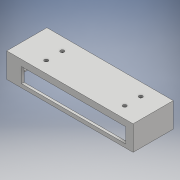
# Autodesk Inventor part: usbhub_holder_new
Saved by Autodesk Inventor 2018 (Build 220112000, 112)
## iProperties
Created: 2019-07-27
Part Number: usbhub_holder_new
Material: 一般
Document SubType Name: Modeling
Designer: guest1
Density: 1 g/cm^3
Appearance: 既定
Author: guest1
Autodesk Inventor part; units mm, degrees
ref_plane "YZ Plane" through (0, 0, 0) normal (1, 0, 0) x (0, 1, 0)
ref_plane "XZ Plane" through (0, 0, 0) normal (0, 1, 0) x (-1, 0, 0)
ref_plane "XY Plane" through (0, 0, 0) normal (0, 0, 1) x (1, 0, 0)
sketch "スケッチ1" plane through (0, 0, 0) normal (0, 0, 1) x (1, 0, 0)
  line L0 (52.125, -16.25) -> (-52.125, -16.25)
  line L1 (-52.125, -16.25) -> (-52.125, 16.25)
  line L2 (-52.125, 16.25) -> (52.125, 16.25)
  line L3 (52.125, 16.25) -> (52.125, -16.25)
  line L4 (52.125, -16.25) -> (-52.125, 16.25) construction
  line L5 (-52.125, -16.25) -> (52.125, 16.25) construction
  point P0 (0, 0)
  dimension "d0" = 104.25
  dimension "d1" = 32.5
  constraints: 12 end point, 2 midpoint, 2 parallel, 1 horizontal, 1 perpendicular
  measures "d0" distance of L1.end L2.end
  measures "d1" distance of L2.end L0.start
extrude "枠" add sketch "スケッチ1" along normal blind 19
sketch "スケッチ2" plane through (0, 0, 0) normal (0, 0, -1) x (-1, 0, 0)
  line L0 (50.125, -14.25) -> (-50.125, -14.25)
  line L1 (-50.125, -14.25) -> (-50.125, 14.25)
  line L2 (-50.125, 14.25) -> (50.125, 14.25)
  line L3 (50.125, 14.25) -> (50.125, -14.25)
  line L4 (50.125, -14.25) -> (-50.125, 14.25) construction
  line L5 (-50.125, -14.25) -> (50.125, 14.25) construction
  point P0 (0, 0)
  dimension "d4" = 100.25
  dimension "d5" = 28.5
  constraints: 12 end point, 2 midpoint, 2 parallel, 1 horizontal, 1 perpendicular
  measures "d4" distance of L1.end L2.end
  measures "d5" distance between parallel lines of L2 L0
extrude "本体" cut sketch "スケッチ2" against normal blind 12
sketch "スケッチ3" plane through (-52.125, -16.25, 0) normal (-1, 0, 0) x (0, 0, 1)
  line L0 (2, 2) -> (14, 2)
  line L1 (14, 2) -> (14, 30.5)
  line L2 (14, 30.5) -> (2, 30.5)
  line L3 (2, 30.5) -> (2, 2)
  line L4 (19, 32.5) -> (19, 0) projected
  line L5 (0, 0) -> (19, 0) projected
  line L6 (0, 0) -> (0, 32.5) projected
  line L7 (0, 32.5) -> (19, 32.5) projected
  point P0 (0, 16.25)
  dimension "d8" = 5
  dimension "d9" = 28.5
  dimension "d10" = 2
  dimension "d11" = 12
  dimension "d12" = 2
  dimension "d13" = 2
  constraints: 8 end point, 2 parallel, 1 horizontal, 1 perpendicular
  measures "d8" distance between parallel lines of L4 L1
  measures "d9" distance of L2.end L0.start
  measures "d10" distance between parallel lines of L5 L0
  measures "d11" distance of L1.end L2.end
  measures "d12" distance between parallel lines of L3 L6
  measures "d13" distance between parallel lines of L7 L2
extrude "入口" cut sketch "スケッチ3" against normal blind 102.25 contours L3 L2 L1 L0
sketch "スケッチ4" plane through (-52.125, -16.25, 0) normal (0, -1, 0) x (1, 0, 0)
  line L0 (98.25, 2) -> (14, 2)
  line L1 (14, 2) -> (14, 14)
  line L2 (14, 14) -> (98.25, 14)
  line L3 (98.25, 14) -> (98.25, 2)
  line L4 (104.25, 0) -> (104.25, 19) projected
  line L5 (0, 0) -> (0, 19) projected
  line L6 (0, 19) -> (104.25, 19) projected
  line L7 (104.25, 0) -> (0, 0) projected
  point P0 (52.125, 0)
  dimension "d16" = 6
  dimension "d17" = 14
  dimension "d18" = 5
  dimension "d19" = 2
  constraints: 8 end point, 2 parallel, 1 horizontal, 1 perpendicular
  measures "d16" distance between parallel lines of L3 L4
  measures "d17" distance between parallel lines of L5 L1
  measures "d18" distance between parallel lines of L6 L2
  measures "d19" distance between parallel lines of L0 L7
extrude "USB穴" cut sketch "スケッチ4" against normal blind 2 contours L0 L1 L2 L3
sketch "スケッチ6" plane through (-52.125, -16.25, 0) normal (-1, 0, 0) x (0, 0, 1)
  line L0 (14, 30.5) -> (14, 2) projected
  line L1 (14, 4) -> (17, 4)
  line L2 (17, 4) -> (17, 13)
  line L3 (17, 13) -> (14, 13)
  line L4 (14, 13) -> (14, 4)
  line L5 (14, 17) -> (17, 17)
  line L6 (17, 17) -> (17, 26)
  line L7 (17, 26) -> (14, 26)
  line L8 (14, 26) -> (14, 17)
  line L9 (14, 2) -> (2, 2) projected
  point P0 (0, 16.25)
  dimension "d22" = 9
  dimension "d23" = 9
  dimension "d24" = 3
  dimension "d25" = 2
  dimension "d26" = 4
  constraints: 16 end point, 4 parallel, 3 point on line, 2 horizontal, 2 perpendicular
  measures "d22" distance of L1.end L2.end
  measures "d23" distance of L5.end L6.end
  measures "d24" distance of L2.end L3.end
  measures "d25" distance between parallel lines of L1 L9
  measures "d26" distance between parallel lines of L5 L3
extrude "ネジ溝" cut sketch "スケッチ6" against normal blind 102.25
sketch "スケッチ7" plane through (-52.125, -12.25, 17) normal (0, 0, -1) x (-1, 0, 0)
  line L0 (-88.25, 5.2069) -> (-24.75, 5.2069)
  line L1 (-24.75, 5.2069) -> (-24.75, 18.2069)
  line L2 (-24.75, 18.2069) -> (-88.25, 18.2069)
  line L3 (-88.25, 18.2069) -> (-88.25, 5.2069)
  line L4 (-104.25, 28.5) -> (-104.25, -4) projected
  point P0 (-52.125, 12.25)
  dimension "d29" = 13
  dimension "d30" = 63.5
  dimension "d31" = 16
  constraints: 8 end point, 2 parallel, 1 horizontal, 1 perpendicular
  measures "d29" distance of L2.end L0.start
  measures "d30" distance of L0.start L0.end
  measures "d31" distance between parallel lines of L3 L4
hole "穴1" at (36.125, -7.0431, 17) at (-27.375, -7.0431, 17) at (-27.375, 5.9569, 17) at (36.125, 5.9569, 17) direction (0, 0, 1) diameter 3 depth 8 tip angle 118
sketch "スケッチ10" plane through (0, 0, 0) normal (0, 0, -1) x (-1, 0, 0)
  line L0 (52.125, -16.25) -> (-52.125, -16.25) projected
  line L1 (-52.125, -16.25) -> (52.125, -16.25)
  line L2 (52.125, -14.25) -> (38.125, -14.25) projected
  line L3 (52.125, 16.25) -> (52.125, -16.25) projected
  line L4 (52.125, -16.25) -> (52.125, 16.25)
  line L5 (-52.125, 16.25) -> (52.125, 16.25) projected
  line L6 (52.125, 16.25) -> (-52.125, 16.25)
  line L7 (-52.125, -16.25) -> (-52.125, 16.25) projected
  line L8 (-52.125, 16.25) -> (-52.125, -16.25)
  line L9 (-48.125, -12.25) -> (48.125, -12.25)
  line L10 (50.125, -14.25) -> (-50.125, -14.25) projected
  line L11 (48.125, -12.25) -> (48.125, 12.25)
  line L12 (48.125, 12.25) -> (-48.125, 12.25)
  line L13 (-48.125, 12.25) -> (-48.125, -12.25)
  point P0 (0, 0)
  dimension "d40" = 4
  dimension "d41" = 4
  dimension "d42" = 4
  dimension "d43" = 4
  constraints: 16 end point, 3 collinear, 2 parallel, 2 perpendicular
  measures "d40" distance between parallel lines of L13 L7
  measures "d41" distance between parallel lines of L0 L9
  measures "d42" distance between parallel lines of L12 L5
  measures "d43" distance between parallel lines of L3 L11
extrude "蓋" add sketch "スケッチ10" along normal blind 1
sketch "スケッチ13" plane through (-52.125, -16.25, 19) normal (-1, 0, 0) x (0, 0, 1)
  line L0 (0, 0) -> (-20, 0) projected
  line L1 (0, 32.5) -> (0, 0) projected
  line L2 (-20, 0) -> (0, 0)
  line L3 (0, 0) -> (0, 32.5)
  line L4 (0, 32.5) -> (-20, 32.5)
  line L5 (-20, 32.5) -> (-20, 0)
  point P0 (-19, 16.25)
  constraints: 8 end point, 2 parallel, 1 horizontal, 1 perpendicular
extrude "調整" cut sketch "スケッチ13" against normal blind 2
